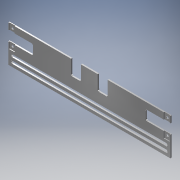
# Autodesk Inventor part: 앞뒷판_위
Saved by Autodesk Inventor 2017 (Build 210142000, 142)
## iProperties
Part Number: 앞뒷판_위
Material: 알루미늄 6061
Document SubType Name: Modeling
Designer: minom
Density: 2.7 g/cm^3
Appearance: 알루미늄 - 평지
Mass: 30.43 g
Surface Area: 130.623 cm^2
Volume: 11.2704 cm^3
Author: minom
Autodesk Inventor part; units mm, degrees
ref_plane "YZ Plane" through (0, 0, 0) normal (1, 0, 0) x (0, 1, 0)
ref_plane "XZ Plane" through (0, 0, 0) normal (0, 1, 0) x (-1, 0, 0)
ref_plane "XY Plane" through (0, 0, 0) normal (0, 0, 1) x (1, 0, 0)
sketch "스케치1" plane through (0, 0, 0) normal (0, 1, 0) x (-1, 0, 0)
  line L0 (0, 0) -> (-230, 0)
  line L1 (-230, 0) -> (-230, 32)
  line L2 (-230, 32) -> (0, 32)
  line L3 (0, 32) -> (0, 0)
  dimension "d0" = 230
  dimension "d1" = 32
  constraints: 8 end point, 2 parallel, 1 horizontal, 1 perpendicular
  measures "d0" distance of L1.end L2.end
  measures "d1" distance of L0.end L1.end
extrude "돌출1" add sketch "스케치1" along normal blind 2
sketch "스케치2" plane through (0, 0, 0) normal (0, -1, 0) x (1, 0, 0)
  line L0 (0, 0) -> (0, 32) projected
  line L1 (230, 0) -> (0, 0) projected
  line L2 (1, 0) -> (1, 32)
  line L3 (0, 32) -> (230, 32) projected
  line L4 (9.2, 32) -> (9.2, 0)
  line L5 (0, 0) -> (230, 0) projected
  line L6 (230, 0) -> (230, 32) projected
  line L7 (230, 32) -> (0, 32) projected
  line L8 (0, 32) -> (0, 0) projected
  line L9 (230, 32) -> (230, 0) projected
  line L10 (230, 32) -> (229, 32)
  line L11 (229, 32) -> (229, 0)
  line L12 (229, 32) -> (220.8, 32)
  line L13 (220.8, 32) -> (220.8, 0)
  line L14 (1, 32) -> (9.2, 32)
  line L15 (1, 0) -> (9.2, 0)
  dimension "d6" = 1
  dimension "d7" = 8.2
  dimension "d10" = 8.2
  dimension "d11" = 1
  constraints: 16 end point, 7 point on line, 2 perpendicular, 1 collinear
  measures "d6" distance of L3.end L10.end
  measures "d7" distance of L10.end L12.end
  measures "d10" distance between parallel lines of L4 L2
  measures "d11" distance between parallel lines of L2 L0
extrude "돌출2" cut sketch "스케치2" against normal blind 1 contours L2 L3 L4 L1 | L13 L3 L11 L1
sketch "스케치3" plane through (0, 2, 0) normal (0, 1, 0) x (1, 0, 0)
  line L0 (230, 0) -> (0, 0) projected
  line L1 (0, 0) -> (0, -32) projected
  line L2 (0, -32) -> (230, -32) projected
  line L3 (230, -32) -> (230, 0) projected
  line L4 (0, -32) -> (230, -32) projected
  line L5 (141, -32) -> (141, -13)
  line L6 (139, -11) -> (129, -11)
  line L7 (127, -13) -> (127, -32)
  line L8 (89, -32) -> (89, -13)
  line L9 (91, -11) -> (101, -11)
  line L10 (103, -13) -> (103, -32)
  arc A0 (103, -13) -> (101, -11) centre (101, -13) ccw
  arc A1 (91, -11) -> (89, -13) centre (91, -13) ccw
  arc A2 (129, -11) -> (127, -13) centre (129, -13) ccw
  arc A3 (141, -13) -> (139, -11) centre (139, -13) ccw
  point P0 (141, -11)
  point P1 (127, -11)
  point P2 (89, -11)
  point P3 (103, -11)
  dimension "d13" = 89
  dimension "d14" = 11
  dimension "d15" = 14
  dimension "d16" = 14
  dimension "d17" = 11
  dimension "d18" = 89
  dimension "d43" = 2
  constraints: 12 end point, 12 point on line, 8 point on circle, 8 tangent, 5 perpendicular, 4 centre point, 3 equal radius
  measures "d13" distance between parallel lines of L3 L5
  measures "d14" distance between parallel lines of L6 L0
  measures "d15" distance between parallel lines of L5 L7
  measures "d16" distance of point (89, -11) point (103, -11)
  measures "d17" distance between parallel lines of L9 L0
  measures "d18" distance between parallel lines of L8 L1
  measures "d43" radius of A0
extrude "돌출3" cut sketch "스케치3" against normal blind 10 contours L2 L7 A2 L6 A3 L5 | L8 A1 L9 A0 L10 L2
sketch "스케치4" plane through (0, 2, 0) normal (0, 1, 0) x (1, 0, 0)
  line L0 (9.2, 0) -> (1, 0) projected
  line L1 (9.2, -32) -> (9.2, 0) projected
  line L2 (1, -32) -> (9.2, -32) projected
  line L3 (1, 0) -> (1, -32) projected
  line L4 (229, -32) -> (229, 0) projected
  line L5 (220.8, -32) -> (229, -32) projected
  line L6 (220.8, 0) -> (220.8, -32) projected
  line L7 (229, 0) -> (220.8, 0) projected
  circle A0 centre (5.1, -5) radius 1.6
  circle A1 centre (5.1, -27) radius 1.6
  circle A2 centre (224.9, -5) radius 1.6
  circle A3 centre (224.9, -27) radius 1.6
  point P0 (0, 0)
  dimension "d21" = 3.2
  dimension "d22" = 3.2
  dimension "d23" = 3.2
  dimension "d24" = 3.2
  dimension "d25" = 4.1
  dimension "d26" = 4.1
  dimension "d27" = 4.1
  dimension "d28" = 4.1
  dimension "d29" = 5
  dimension "d30" = 5
  dimension "d31" = 5
  dimension "d32" = 5
  constraints: 4 centre point
  measures "d21" diameter of A0
  measures "d22" diameter of A1
  measures "d23" diameter of A2
  measures "d24" diameter of A3
  measures "d25" distance from line of L3 A0.centre
  measures "d26" distance from line of L3 A1.centre
  measures "d27" distance from line of L6 A3.centre
  measures "d28" distance from line of L4 A2.centre
  measures "d29" distance from line of L7 A2.centre
  measures "d30" distance from line of L5 A3.centre
  measures "d31" distance from line of L0 A0.centre
  measures "d32" distance from line of L2 A1.centre
extrude "돌출4" cut sketch "스케치4" against normal blind 10 contours A0 | A1 | A2 | A3
sketch "스케치5" plane through (0, 2, 0) normal (0, 1, 0) x (1, 0, 0)
  circle A0 centre (224.9, -5) radius 1.6 projected
  circle A1 centre (5.1, -5) radius 1.6 projected
  circle A2 centre (5.1, -27) radius 1.6 projected
  circle A3 centre (224.9, -27) radius 1.6 projected
  line L0 (141, -13) -> (141, -32) projected
  line L1 (141, -32) -> (230, -32) projected
  line L2 (230, -32) -> (230, 0) projected
  line L3 (230, 0) -> (0, 0) projected
  line L4 (0, 0) -> (0, -32) projected
  line L5 (0, -32) -> (89, -32) projected
  line L6 (89, -32) -> (89, -13) projected
  line L7 (91, -11) -> (101, -11) projected
  line L8 (103, -13) -> (103, -32) projected
  line L9 (103, -32) -> (127, -32) projected
  line L10 (127, -32) -> (127, -13) projected
  line L11 (129, -11) -> (139, -11) projected
  line L12 (230, -32) -> (230, 0) projected
  line L13 (230, -9) -> (197, -9)
  line L14 (195, -11) -> (195, -21)
  line L15 (197, -23) -> (230, -23)
  line L16 (230, -23) -> (230, -9)
  line L17 (0, 0) -> (0, -32) projected
  line L18 (0, -9) -> (33, -9)
  line L19 (35, -11) -> (35, -21)
  line L20 (33, -23) -> (0, -23)
  line L21 (0, -23) -> (0, -9)
  arc A4 (129, -11) -> (127, -13) centre (129, -13) ccw projected
  arc A5 (141, -13) -> (139, -11) centre (139, -13) ccw projected
  arc A6 (91, -11) -> (89, -13) centre (91, -13) ccw projected
  arc A7 (103, -13) -> (101, -11) centre (101, -13) ccw projected
  arc A8 (195, -21) -> (197, -23) centre (197, -21) ccw
  arc A9 (197, -9) -> (195, -11) centre (197, -11) ccw
  arc A10 (33, -23) -> (35, -21) centre (33, -21) ccw
  arc A11 (35, -11) -> (33, -9) centre (33, -11) ccw
  point P0 (195, -23)
  point P1 (195, -9)
  point P2 (35, -23)
  point P3 (35, -9)
  dimension "d35" = 35
  dimension "d36" = 14
  dimension "d37" = 9
  dimension "d38" = 35
  dimension "d39" = 14
  dimension "d40" = 9
  dimension "d44" = 2
  constraints: 16 end point, 10 point on line, 8 point on circle, 8 tangent, 4 centre point, 4 parallel, 3 equal radius, 2 horizontal, 2 perpendicular
  measures "d35" distance of L15.end point (195, -23)
  measures "d36" distance of point (195, -23) point (195, -9)
  measures "d37" distance between parallel lines of L13 L3
  measures "d38" distance of point (35, -23) L20.end
  measures "d39" distance of point (35, -9) point (35, -23)
  measures "d40" distance between parallel lines of L18 L3
  measures "d44" radius of A8
extrude "돌출5" cut sketch "스케치5" against normal blind 10 contours L15 A8 L14 A9 L13 L2 | L18 A11 L19 A10 L20 L4
sketch "스케치6" plane through (0, 2, 0) normal (0, 1, 0) x (1, 0, 0)
  circle A0 centre (224.9, -27) radius 1.6 projected
  circle A1 centre (5.1, -27) radius 1.6 projected
  circle A2 centre (5.1, -5) radius 1.6 projected
  circle A3 centre (224.9, -5) radius 1.6 projected
  line L0 (230, -23) -> (197, -23) projected
  arc A4 (195, -21) -> (197, -23) centre (197, -21) ccw projected
  line L1 (195, -21) -> (195, -11) projected
  arc A5 (197, -9) -> (195, -11) centre (197, -11) ccw projected
  line L2 (197, -9) -> (230, -9) projected
  line L3 (230, -9) -> (230, 0) projected
  line L4 (230, 0) -> (0, 0) projected
  line L5 (0, 0) -> (0, -9) projected
  line L6 (0, -9) -> (33, -9) projected
  arc A6 (35, -11) -> (33, -9) centre (33, -11) ccw projected
  line L7 (35, -11) -> (35, -21) projected
  arc A7 (33, -23) -> (35, -21) centre (33, -21) ccw projected
  line L8 (33, -23) -> (0, -23) projected
  line L9 (0, -23) -> (0, -32) projected
  line L10 (0, -32) -> (89, -32) projected
  line L11 (89, -32) -> (89, -13) projected
  arc A8 (91, -11) -> (89, -13) centre (91, -13) ccw projected
  line L12 (91, -11) -> (101, -11) projected
  arc A9 (103, -13) -> (101, -11) centre (101, -13) ccw projected
  line L13 (103, -13) -> (103, -32) projected
  line L14 (103, -32) -> (127, -32) projected
  line L15 (127, -32) -> (127, -13) projected
  arc A10 (129, -11) -> (127, -13) centre (129, -13) ccw projected
  line L16 (129, -11) -> (139, -11) projected
  arc A11 (141, -13) -> (139, -11) centre (139, -13) ccw projected
  line L17 (141, -13) -> (141, -32) projected
  line L18 (141, -32) -> (230, -32) projected
  line L19 (230, -32) -> (230, -23) projected
  line L20 (0, 0) -> (230, 0)
  line L21 (230, 0) -> (230, 20)
  line L22 (230, 20) -> (0, 20)
  line L23 (0, 20) -> (0, 0)
  line L24 (6, 16) -> (224, 16)
  line L25 (224, 12) -> (6, 12)
  line L26 (6, 8) -> (224, 8)
  line L27 (224, 4) -> (6, 4)
  arc A12 (224, 4) -> (224, 8) centre (224, 6) ccw
  arc A13 (224, 12) -> (224, 16) centre (224, 14) ccw
  arc A14 (6, 16) -> (6, 12) centre (6, 14) ccw
  arc A15 (6, 8) -> (6, 4) centre (6, 6) ccw
  dimension "d45" = 230
  dimension "d46" = 20
  dimension "d47" = 4
  dimension "d48" = 4
  dimension "d51" = 4
  dimension "d52" = 4
  dimension "d57" = 6
  dimension "d58" = 2
  dimension "d59" = 2
  dimension "d61" = 2
  dimension "d62" = 2
  dimension "d63" = 6
  dimension "d64" = 2
  dimension "d65" = 2
  dimension "d66" = 6
  dimension "d67" = 6
  dimension "d68" = 6
  dimension "d69" = 6
  constraints: 16 end point, 8 point on circle, 4 centre point, 4 parallel, 3 horizontal, 1 perpendicular
  measures "d45" distance of L22.end L21.end
  measures "d46" distance of L21.end L20.end
  measures "d47" distance between parallel lines of L24 L22
  measures "d48" distance between parallel lines of L25 L24
  measures "d51" distance between parallel lines of L27 L26
  measures "d52" distance between parallel lines of L25 L26
  measures "d57" distance from line of L21 A12.centre
  measures "d58" radius of A12
  measures "d59" distance from line of L26 A12.centre
  measures "d61" distance from line of L24 A13.centre
  measures "d62" radius of A13
  measures "d63" distance from line of L21 A13.centre
  measures "d64" radius of A14
  measures "d65" radius of A15
  measures "d66" distance from line of L22 A14.centre
  measures "d67" distance from line of L23 A14.centre
  measures "d68" distance from line of L4 A15.centre
  measures "d69" distance from line of L23 A15.centre
extrude "돌출6" add sketch "스케치6" against normal blind 2 contours L4 L23 L22 L21
